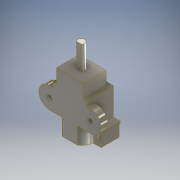
# Autodesk Inventor part: Motor
Saved by Autodesk Inventor 2017 (Build 210142000, 142)
## iProperties
Part Number: Motor
Material: Titanio
Document SubType Name: Modeling
Designer: fam
Density: 4.51 g/cm^3
Appearance: Plata
Author: fam
Autodesk Inventor part; units mm, degrees
ref_plane "YZ Plane" through (0, 0, 0) normal (1, 0, 0) x (0, 1, 0)
ref_plane "XZ Plane" through (0, 0, 0) normal (0, 1, 0) x (-1, 0, 0)
ref_plane "XY Plane" through (0, 0, 0) normal (0, 0, 1) x (1, 0, 0)
sketch "Boceto1" plane through (0, 0, 0) normal (0, 0, 1) x (1, 0, 0)
  circle A0 centre (0, 0) radius 1.5
  line L0 (-1.118, -1) -> (1.118, -1)
  dimension "d0" = 3
  dimension "d1" = 2.5
  constraints: 2 end point, 2 point on circle, 1 centre point, 1 coincident, 1 horizontal
  measures "d0" diameter of A0
extrude "Extrusión1" add sketch "Boceto1" against normal blind 10.58 contours A0 L0 picked at (0.0594, -0.1702)
sketch "Boceto2" plane through (0, 0, -10.58) normal (0, 0, -1) x (-1, 0, 0)
  line L0 (-6, 5) -> (6, 5)
  line L1 (6, 5) -> (6, -5)
  line L2 (6, -5) -> (-6, -5)
  line L3 (-6, -5) -> (-6, 5)
  point P0 (0, 0)
  dimension "d4" = 10
  dimension "d5" = 12
  dimension "d6" = 5
  dimension "d7" = 6
  constraints: 8 end point, 2 horizontal, 2 vertical
  measures "d4" distance of L0.end L1.end
  measures "d5" distance of L0.start L0.end
  measures "d6" distance from line of L0 point (0, 0)
  measures "d7" distance from line of L1 point (0, 0)
extrude "Extrusión2" add sketch "Boceto2" along normal blind 6
sketch "Boceto3" plane through (0, 0, -16.58) normal (0, 0, -1) x (-1, 0, 0)
  line L0 (-7.5, 6.77) -> (7.5, 6.77)
  line L1 (7.5, 6.77) -> (7.5, -5)
  line L2 (7.5, -5) -> (-7.5, -5)
  line L3 (-7.5, -5) -> (-7.5, 6.77)
  line L4 (-6, -5) -> (6, -5) projected
  point P0 (0, 0)
  point P1 (0, -5)
  dimension "d10" = 15
  dimension "d11" = 11.77
  constraints: 8 end point, 2 horizontal, 2 midpoint, 2 vertical, 1 horizontal alignment
  measures "d10" distance of L0.start L0.end
  measures "d11" distance of L0.end L1.end
extrude "Extrusión3" add sketch "Boceto3" along normal blind 11.77
sketch "Boceto4" plane through (-6, -5, -10.58) normal (0, -1, 0) x (1, 0, 0)
  circle A0 centre (15, -13) radius 1
  circle A1 centre (-3, -13) radius 1
  circle A2 centre (-3, -13) radius 4.77
  circle A3 centre (15, -13) radius 4.77
  line L0 (-1.5, -6) -> (0, -6) projected
  line L1 (13.5, -17.77) -> (-1.5, -17.77) projected
  line L2 (15, -17.77) -> (-3, -17.77)
  line L3 (15, -8.23) -> (-3, -8.23)
  point P0 (6, 10.58)
  dimension "d14" = 2
  dimension "d15" = 18
  dimension "d16" = 9
  dimension "d18" = 7
  constraints: 4 centre point, 4 end point, 4 point on circle, 3 tangent, 2 concentric, 2 equal radius, 2 horizontal, 1 horizontal alignment
  measures "d14" diameter of A0
  measures "d15" distance of A1.centre A0.centre
  measures "d16" horizontal distance of point (6, 10.58) A1.centre
  measures "d18" distance from line of L0 A1.centre
extrude "Extrusión4" add sketch "Boceto4" against normal blind 3
sketch "Boceto5" plane through (0, 0, -28.35) normal (0, 0, -1) x (-1, 0, 0)
  circle A0 centre (0, 0) radius 6
  line L0 (-3.3166, 5) -> (3.3166, 5)
  line L1 (-3.3166, -5) -> (3.3166, -5)
  line L2 (9, -5) -> (-9, -5) projected
  point P0 (0, -5)
  dimension "d21" = 12
  constraints: 4 end point, 4 point on circle, 2 horizontal, 2 midpoint, 1 centre point, 1 coincident, 1 vertical alignment
  measures "d21" diameter of A0
extrude "Extrusión5" add sketch "Boceto5" along normal blind 7.33 contours A0 L1 L0
sketch "Boceto6" plane through (0, 0, -35.68) normal (0, 0, -1) x (-1, 0, 0)
  line L0 (-4.5, 12.8) -> (4.5, 12.8)
  line L1 (4.5, 12.8) -> (4.5, 3.9686)
  line L2 (4.5, 3.9686) -> (-4.5, 3.9686)
  line L3 (-4.5, 3.9686) -> (-4.5, 12.8)
  line L4 (-3.3166, -5) -> (3.3166, -5) projected
  arc A0 (3.3166, -5) -> (3.3166, 5) centre (0, 0) ccw projected
  point P0 (0, 12.8)
  dimension "d24" = 9
  dimension "d25" = 17.8
  constraints: 8 end point, 2 horizontal, 2 vertical, 1 midpoint, 1 point on circle, 1 vertical alignment
  measures "d24" distance of L0.start L0.end
  measures "d25" distance between parallel lines of L4 L0
extrude "Extrusión6" add sketch "Boceto6" against normal blind 1
sketch "Boceto7" plane through (0, 0, -35.68) normal (0, 0, -1) x (-1, 0, 0)
  line L0 (-4, 12.8) -> (4, 12.8)
  line L1 (4, 12.8) -> (4, 4.8)
  line L2 (4, 4.8) -> (-4, 4.8)
  line L3 (-4, 4.8) -> (-4, 12.8)
  line L4 (-4.5, 12.8) -> (4.5, 12.8) projected
  point P0 (0, 0)
  point P1 (0, 12.8)
  dimension "d28" = 8
  dimension "d29" = 8
  constraints: 8 end point, 2 horizontal, 2 midpoint, 2 vertical, 1 vertical alignment
  measures "d28" distance of L0.start L0.end
  measures "d29" distance of L0.end L1.end
extrude "Extrusión7" add sketch "Boceto7" along normal blind 5.5
shell "Vaciado1" thickness 1 removed faces 1 at (1.3333, 12.8, -39.3467)
